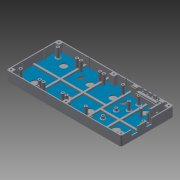
# Autodesk Inventor part: bottom-cover
Saved by Autodesk Inventor 2015 (Build 190159000, 159)
## iProperties
Created: 2016-04-25
Part Number: bottom-cover
Material: 一般
Document SubType Name: Modeling
Designer: yamashita1
Density: 1 g/cm^3
Appearance: 既定
Author: yamashita1
Autodesk Inventor part; units mm, degrees
ref_plane "YZ Plane" through (0, 0, 0) normal (1, 0, 0) x (0, 1, 0)
ref_plane "XZ Plane" through (0, 0, 0) normal (0, 1, 0) x (-1, 0, 0)
ref_plane "XY Plane" through (0, 0, 0) normal (0, 0, 1) x (1, 0, 0)
sketch "スケッチ1" plane through (0, 0, 0) normal (0, 0, 1) x (1, 0, 0)
  line L0 (-120, 55) -> (120, 55)
  line L1 (120, 55) -> (120, -55)
  line L2 (120, -55) -> (-120, -55)
  line L3 (-120, -55) -> (-120, 55)
  point P0 (0, 0)
  dimension "d0" = 240
  dimension "d1" = 110
  dimension "d2" = 120
  dimension "d3" = 55
  constraints: 8 end point, 2 parallel, 1 horizontal, 1 perpendicular
  measures "d0" distance of L1.end L2.end
  measures "d1" distance of L0.end L1.end
  measures "d2" distance from line of L3 point (0, 0)
  measures "d3" distance from line of L2 point (0, 0)
extrude "底" add sketch "スケッチ1" along normal blind 20
sketch "スケッチ2" plane through (0, 0, 20) normal (0, 0, 1) x (1, 0, 0)
  line L0 (-118, 53) -> (118, 53)
  line L1 (118, 53) -> (118, -53)
  line L2 (118, -53) -> (-118, -53)
  line L3 (-118, -53) -> (-118, 53)
  point P0 (0, 0)
  dimension "d6" = 236
  dimension "d7" = 106
  dimension "d8" = 118
  dimension "d9" = 53
  constraints: 8 end point, 2 parallel, 1 horizontal, 1 perpendicular
  measures "d6" distance of L1.end L2.end
  measures "d7" distance of L0.end L1.end
  measures "d8" distance from line of L3 point (0, 0)
  measures "d9" distance from line of L2 point (0, 0)
extrude "底 くりぬき" cut sketch "スケッチ2" against normal blind 18
sketch "スケッチ3" plane through (0, 0, 2) normal (0, 0, 1) x (1, 0, 0)
  line L0 (-118, 53) -> (-110, 53)
  line L1 (-110, 53) -> (-110, 45)
  line L2 (-110, 45) -> (-118, 45)
  line L3 (-118, 45) -> (-118, 53)
  line L4 (-118, -53) -> (-110, -53)
  line L5 (-110, -53) -> (-110, -45)
  line L6 (-110, -45) -> (-118, -45)
  line L7 (-118, -45) -> (-118, -53)
  line L8 (118, -53) -> (110, -53)
  line L9 (110, -53) -> (110, -45)
  line L10 (110, -45) -> (118, -45)
  line L11 (118, -45) -> (118, -53)
  line L12 (118, 53) -> (110, 53)
  line L13 (110, 53) -> (110, 45)
  line L14 (110, 45) -> (118, 45)
  line L15 (118, 45) -> (118, 53)
  line L16 (-5, 53) -> (5, 53)
  line L17 (5, 53) -> (5, 45)
  line L18 (5, 45) -> (-5, 45)
  line L19 (-5, 45) -> (-5, 53)
  line L20 (-5, -45) -> (5, -45)
  line L21 (5, -45) -> (5, -53)
  line L22 (5, -53) -> (-5, -53)
  line L23 (-5, -53) -> (-5, -45)
  line L24 (118, -53) -> (-118, -53) projected
  line L25 (-118, 53) -> (118, 53) projected
  point P0 (0, 0)
  point P1 (0, 45)
  point P2 (0, -53)
  point P3 (0, -53)
  point P4 (0, 53)
  dimension "d13" = 8
  dimension "d14" = 8
  dimension "d15" = 8
  dimension "d16" = 8
  dimension "d17" = 8
  dimension "d18" = 8
  dimension "d19" = 8
  dimension "d117" = 8
  dimension "d161" = 10
  dimension "d162" = 8
  dimension "d165" = 10
  dimension "d166" = 8
  constraints: 48 end point, 12 parallel, 6 horizontal, 6 perpendicular, 4 midpoint, 2 collinear, 2 vertical alignment, 1 coincident
  measures "d13" distance of L0.end L1.end
  measures "d14" distance of L6.end L5.end
  measures "d15" distance of L5.end L4.end
  measures "d16" distance of L9.end L10.end
  measures "d17" distance of L8.end L9.end
  measures "d18" distance of L14.end L13.end
  measures "d19" distance of L13.end L12.end
  measures "d117" distance from line of L3 L1.end
  measures "d161" distance of L17.end L18.end
  measures "d162" distance of L16.end L17.end
  measures "d165" distance of L21.end L22.end
  measures "d166" distance of L20.end L21.end
extrude "天板固定用ボス" add sketch "スケッチ3" along normal blind 18
sketch "スケッチ4" plane through (0, 0, 20) normal (0, 0, 1) x (1, 0, 0)
  circle A0 centre (-115, 50) radius 1.6
  line L0 (-120, 55) -> (-120, -55) projected
  line L1 (120, 55) -> (-120, 55) projected
  circle A1 centre (-115, -50) radius 1.6
  line L2 (-120, -55) -> (120, -55) projected
  circle A2 centre (115, 50) radius 1.6
  line L3 (120, -55) -> (120, 55) projected
  circle A3 centre (115, -50) radius 1.6
  circle A4 centre (0, 50) radius 1.6
  circle A5 centre (0, -50) radius 1.6
  point P0 (0, 0)
  dimension "d22" = 3.2
  dimension "d23" = 5
  dimension "d24" = 5
  dimension "d25" = 3.2
  dimension "d26" = 5
  dimension "d27" = 5
  dimension "d28" = 3.2
  dimension "d29" = 5
  dimension "d30" = 5
  dimension "d31" = 3.2
  dimension "d32" = 5
  dimension "d33" = 5
  constraints: 6 centre point, 2 equal radius, 2 horizontal alignment, 2 vertical alignment
  measures "d22" diameter of A0
  measures "d23" distance from line of L0 A0.centre
  measures "d24" distance from line of L1 A0.centre
  measures "d25" diameter of A1
  measures "d26" distance from line of L0 A1.centre
  measures "d27" distance from line of L2 A1.centre
  measures "d28" diameter of A2
  measures "d29" distance from line of L1 A2.centre
  measures "d30" distance from line of L3 A2.centre
  measures "d31" diameter of A3
  measures "d32" distance from line of L3 A3.centre
  measures "d33" distance from line of L2 A3.centre
extrude "天板固定用穴" cut sketch "スケッチ4" against normal blind 20 contours A0 | A1 | A2 | A3 | A4 | A5
sketch "スケッチ5" plane through (0, 0, 0) normal (0, 0, -1) x (-1, 0, 0)
  circle A0 centre (115, -50) radius 3.5
  circle A1 centre (115, -50) radius 1.6 projected
  circle A2 centre (115, 50) radius 3.5
  circle A3 centre (115, 50) radius 1.6 projected
  circle A4 centre (-115, 50) radius 3.5
  circle A5 centre (-115, 50) radius 1.6 projected
  circle A6 centre (-115, -50) radius 3.5
  circle A7 centre (-115, -50) radius 1.6 projected
  circle A8 centre (0, -50) radius 1.6 projected
  circle A9 centre (0, -50) radius 3.5
  circle A10 centre (0, 50) radius 1.6 projected
  circle A11 centre (0, 50) radius 3.5
  point P0 (0, 0)
  dimension "d39" = 7
  constraints: 6 centre point, 5 equal radius, 4 concentric, 2 coincident
  measures "d39" diameter of A6
extrude "天板固定用穴ザグリ" cut sketch "スケッチ5" against normal blind 15
sketch "スケッチ6" plane through (0, 0, 2) normal (0, 0, 1) x (1, 0, 0)
  circle A0 centre (-10, -39) radius 3.25
  circle A1 centre (-10, 39) radius 3.25
  circle A2 centre (30, 39) radius 3.25
  circle A3 centre (30, -39) radius 3.25
  point P0 (0, 0)
  dimension "d42" = 39
  dimension "d43" = 10
  dimension "d44" = 40
  dimension "d45" = 39
  dimension "d46" = 6.5
  dimension "d47" = 6.5
  dimension "d48" = 6.5
  dimension "d49" = 6.5
  constraints: 4 centre point, 4 coincident, 2 horizontal alignment, 2 vertical alignment
  measures "d42" vertical distance of point (-10, -39) point (0, 0)
  measures "d43" horizontal distance of point (-10, -39) point (0, 0)
  measures "d44" distance of point (30, -39) point (-10, -39)
  measures "d45" vertical distance of point (-10, 39) point (0, 0)
  measures "d46" diameter of A0
  measures "d47" diameter of A1
  measures "d48" diameter of A2
  measures "d49" diameter of A3
extrude "7セグ固定用ボス" add sketch "スケッチ6" along normal blind 19.4
sketch "スケッチ7" plane through (-10, 39, 21.4) normal (0, 0, 1) x (1, 0, 0)
  circle A0 centre (0, 0) radius 1.4
  circle A1 centre (0, 0) radius 3.25 projected
  circle A2 centre (0, -78) radius 1.4
  circle A3 centre (0, -78) radius 3.25 projected
  circle A4 centre (40, 0) radius 1.4
  circle A5 centre (40, 0) radius 3.25 projected
  circle A6 centre (40, -78) radius 1.4
  circle A7 centre (40, -78) radius 3.25 projected
  point P0 (10, -39)
  dimension "d52" = 2.8
  dimension "d53" = 2.8
  dimension "d54" = 2.8
  dimension "d55" = 2.8
  constraints: 4 centre point, 4 concentric
  measures "d52" diameter of A0
  measures "d53" diameter of A2
  measures "d54" diameter of A4
  measures "d55" diameter of A6
extrude "7セグ固定用ボス ねじ穴" cut sketch "スケッチ7" against normal blind 10 contours A0 | A2 | A4 | A6
pattern_linear "矩形状パターン1" count 3 spacing 48 along (-1, 0, 0) of "7セグ固定用ボス", "7セグ固定用ボス ねじ穴"
sketch "スケッチ8" plane through (120, -55, 0) normal (1, 0, 0) x (0, 0, -1)
  line L0 (-20, 110) -> (-20, 0) projected
  line L1 (-20, 53.38) -> (-9, 53.38)
  line L2 (-9, 53.38) -> (-9, 64.38)
  line L3 (-9, 64.38) -> (-20, 64.38)
  line L4 (-20, 64.38) -> (-20, 53.38)
  line L5 (-20, 21.9) -> (-9, 21.9)
  line L6 (-9, 21.9) -> (-9, 34.9)
  line L7 (-9, 34.9) -> (-20, 34.9)
  line L8 (-20, 34.9) -> (-20, 21.9)
  line L9 (-20, 0) -> (-20, 110) projected
  point P0 (0, 55)
  point P1 (-20, 66.5)
  point P2 (-20, 58.88)
  point P3 (-20, 28.4)
  point P4 (-20, 58.88)
  point P5 (-20, 28.4)
  dimension "d197" = 11.5
  dimension "d198" = 7.62
  dimension "d199" = 38.1
  dimension "d200" = 11
  dimension "d201" = 11
  dimension "d202" = 11
  dimension "d203" = 13
  constraints: 16 end point, 4 parallel, 3 point on line, 2 coincident, 2 collinear, 2 horizontal, 2 midpoint, 2 perpendicular
  measures "d197" vertical distance of point (0, 55) point (-20, 66.5)
  measures "d198" distance of point (-20, 58.88) point (-20, 66.5)
  measures "d199" distance of point (-20, 28.4) point (-20, 66.5)
  measures "d200" distance of L3.end L2.end
  measures "d201" distance of L2.end L1.end
  measures "d202" distance of L7.end L6.end
  measures "d203" distance of L6.end L5.end
extrude "Arduinoコネクタ穴" cut sketch "スケッチ8" against normal blind 2
sketch "スケッチ9" plane through (0, 0, 2) normal (0, 0, 1) x (1, 0, 0)
  line L0 (118, 45) -> (118, -45) projected
  circle A0 centre (103.03, 8.96) radius 3
  circle A1 centre (50.96, 3.88) radius 3
  circle A2 centre (50.96, -24.06) radius 3
  circle A3 centre (101.76, -39.3) radius 3
  point P0 (0, 0)
  point P1 (118, 11.5)
  point P2 (118, 8.88)
  dimension "d75" = 11.5
  dimension "d76" = 14.97
  dimension "d77" = 2.54
  dimension "d78" = 67.04
  dimension "d79" = 7.62
  dimension "d80" = 27.94
  dimension "d81" = 16.24
  dimension "d82" = 50.8
  dimension "d83" = 6
  constraints: 4 centre point, 4 coincident, 3 equal radius, 1 point on line, 1 vertical alignment
  measures "d75" vertical distance of point (118, 11.5) point (0, 0)
  measures "d76" horizontal distance of point (103.03, 8.96) point (118, 11.5)
  measures "d77" vertical distance of point (103.03, 8.96) point (118, 11.5)
  measures "d78" horizontal distance of point (50.96, 3.88) point (118, 11.5)
  measures "d79" vertical distance of point (50.96, 3.88) point (118, 11.5)
  measures "d80" distance of point (50.96, -24.06) point (50.96, 3.88)
  measures "d81" horizontal distance of point (101.76, -39.3) point (118, 11.5)
  measures "d82" vertical distance of point (101.76, -39.3) point (118, 11.5)
  measures "d83" diameter of A0
extrude "Arduino固定用ボス" add sketch "スケッチ9" along normal blind 5.2
sketch "スケッチ10" plane through (103.03, 8.96, 7.2) normal (0, 0, 1) x (1, 0, 0)
  circle A0 centre (0, 0) radius 1.4
  circle A1 centre (0, 0) radius 3 projected
  circle A2 centre (-52.07, -5.08) radius 1.4
  circle A3 centre (-52.07, -33.02) radius 1.4
  circle A4 centre (-52.07, -5.08) radius 3 projected
  circle A5 centre (-52.07, -33.02) radius 3 projected
  point P0 (-103.03, -8.96)
  dimension "d86" = 2.8
  constraints: 3 centre point, 3 concentric, 2 equal radius
  measures "d86" diameter of A0
extrude "Arduino固定用ボス ねじ穴" cut sketch "スケッチ10" against normal blind 5.2 contours A0 | A2 | A3
sketch "スケッチ11" plane through (-120, 55, 0) normal (0, 1, 0) x (1, 0, 0)
  line L0 (230, -20) -> (10, -20) projected
  line L1 (209.24, -20) -> (205.24, -20)
  line L2 (205.24, -20) -> (205.24, -14.5)
  line L3 (205.24, -14.5) -> (209.24, -14.5)
  line L4 (209.24, -14.5) -> (209.24, -20)
  line L5 (240, -20) -> (0, -20) projected
  point P0 (120, 0)
  point P1 (192, -20)
  point P2 (207.24, -20)
  point P3 (207.24, -14.5)
  dimension "d89" = 72
  dimension "d90" = 15.24
  dimension "d91" = 4
  dimension "d92" = 5.5
  constraints: 8 end point, 2 parallel, 2 point on line, 1 collinear, 1 horizontal, 1 midpoint, 1 perpendicular, 1 vertical alignment
  measures "d89" horizontal distance of point (192, -20) point (120, 0)
  measures "d90" distance of point (207.24, -20) point (192, -20)
  measures "d91" distance of L2.end L3.end
  measures "d92" distance of L1.end L2.end
extrude "タクトスイッチ穴" cut sketch "スケッチ11" against normal blind 2
pattern_linear "矩形状パターン2" count 4 spacing 10.16 along (-1, 0, 0) of "タクトスイッチ穴"
sketch "スケッチ12" plane through (0, 0, 2) normal (0, 0, 1) x (1, 0, 0)
  line L0 (-110, 53) -> (110, 53) projected
  line L1 (40, 53) -> (104, 53)
  line L2 (104, 53) -> (104, 45)
  line L3 (104, 45) -> (40, 45)
  line L4 (40, 45) -> (40, 53)
  line L5 (68.92, 53) -> (75.08, 53) projected
  line L6 (89.24, 53) -> (110, 53) projected
  point P0 (0, 0)
  point P1 (72, 53)
  point P2 (72, 45)
  point P3 (72, 53)
  dimension "d98" = 72
  dimension "d99" = 64
  dimension "d100" = 8
  constraints: 8 end point, 2 midpoint, 2 parallel, 1 collinear, 1 horizontal, 1 perpendicular, 1 point on line, 1 vertical alignment
  measures "d98" horizontal distance of point (72, 53) point (0, 0)
  measures "d99" distance of L2.end L3.end
  measures "d100" distance of L1.end L2.end
extrude "タクトスイッチ固定用ボス" add sketch "スケッチ12" along normal blind 18
sketch "スケッチ13" plane through (0, 0, 20) normal (0, 0, 1) x (1, 0, 0)
  line L0 (75.08, 55) -> (68.92, 55) projected
  line L1 (42, 48) -> (102, 48)
  line L2 (102, 48) -> (102, 46.2)
  line L3 (102, 46.2) -> (42, 46.2)
  line L4 (42, 46.2) -> (42, 48)
  point P0 (0, 0)
  point P1 (72, 55)
  point P2 (72, 46.2)
  point P3 (72, 55)
  dimension "d103" = 60
  dimension "d104" = 1.8
  dimension "d105" = 7
  constraints: 8 end point, 3 midpoint, 2 parallel, 1 horizontal, 1 perpendicular, 1 vertical alignment
  measures "d103" distance of L2.end L3.end
  measures "d104" distance of L1.end L2.end
  measures "d105" vertical distance of L1.start point (72, 55)
extrude "タクトスイッチ基板用スリット" cut sketch "スケッチ13" against normal blind 11
sketch "スケッチ14" plane through (0, 0, 20) normal (0, 0, 1) x (1, 0, 0)
  line L0 (75.08, 55) -> (68.92, 55) projected
  line L1 (49.5, 53) -> (94.5, 53)
  line L2 (94.5, 53) -> (94.5, 48)
  line L3 (94.5, 48) -> (49.5, 48)
  line L4 (49.5, 48) -> (49.5, 53)
  point P0 (0, 0)
  point P1 (72, 55)
  point P2 (72, 48)
  point P3 (72, 55)
  dimension "d108" = 45
  dimension "d109" = 5
  dimension "d110" = 2
  constraints: 8 end point, 3 midpoint, 2 parallel, 1 horizontal, 1 perpendicular, 1 vertical alignment
  measures "d108" distance of L2.end L3.end
  measures "d109" distance of L1.end L2.end
  measures "d110" vertical distance of L1.start point (72, 55)
extrude "タクトスイッチ基板用くりぬき1" cut sketch "スケッチ14" against normal blind 6.8
sketch "スケッチ15" plane through (0, 0, 20) normal (0, 0, 1) x (1, 0, 0)
  line L0 (75.08, 55) -> (68.92, 55) projected
  line L1 (49.5, 45) -> (94.5, 45)
  line L2 (94.5, 45) -> (94.5, 47.5)
  line L3 (94.5, 47.5) -> (49.5, 47.5)
  line L4 (49.5, 47.5) -> (49.5, 45)
  line L5 (40, 45) -> (104, 45) projected
  point P0 (0, 0)
  point P1 (72, 55)
  point P2 (72, 45)
  point P3 (72, 55)
  dimension "d113" = 45
  dimension "d114" = 2.5
  constraints: 8 end point, 3 midpoint, 2 parallel, 1 collinear, 1 horizontal, 1 perpendicular, 1 vertical alignment
  measures "d113" distance of L3.end L2.end
  measures "d114" distance of L2.end L1.end
extrude "タクトスイッチ基板用くりぬき2" cut sketch "スケッチ15" against normal blind 7.5
sketch "スケッチ16" plane through (0, 0, 2) normal (0, 0, 1) x (1, 0, 0)
  circle A0 centre (104.32, 38.16) radius 3
  circle A1 centre (63.68, 38.16) radius 3
  circle A2 centre (63.68, 17.84) radius 3
  circle A3 centre (104.32, 17.84) radius 3
  circle A4 centre (89.08, 17.84) radius 2.5
  point P0 (0, 0)
  point P1 (84, 28)
  dimension "d118" = 84
  dimension "d119" = 28
  dimension "d120" = 20.32
  dimension "d121" = 10.16
  dimension "d122" = 20.32
  dimension "d123" = 10.16
  dimension "d124" = 6
  dimension "d125" = 5.08
  dimension "d126" = 5
  constraints: 5 centre point, 5 coincident, 3 equal radius, 3 horizontal alignment, 2 vertical alignment
  measures "d118" horizontal distance of point (84, 28) point (0, 0)
  measures "d119" vertical distance of point (0, 0) point (84, 28)
  measures "d120" horizontal distance of point (104.32, 38.16) point (84, 28)
  measures "d121" vertical distance of point (84, 28) point (104.32, 38.16)
  measures "d122" horizontal distance of point (84, 28) point (63.68, 38.16)
  measures "d123" vertical distance of point (104.32, 17.84) point (84, 28)
  measures "d124" diameter of A0
  measures "d125" horizontal distance of point (84, 28) point (89.08, 17.84)
  measures "d126" diameter of A4
extrude "LCD RTC基板固定用ボス" add sketch "スケッチ16" along normal blind 16.7
sketch "スケッチ17" plane through (104.32, 38.16, 18.7) normal (0, 0, 1) x (1, 0, 0)
  circle A0 centre (0, 0) radius 1.4
  circle A1 centre (-40.64, 0) radius 1.4
  circle A2 centre (-40.64, -20.32) radius 1.4
  circle A3 centre (0, -20.32) radius 1.4
  circle A4 centre (0, 0) radius 3 projected
  circle A5 centre (-40.64, 0) radius 3 projected
  circle A6 centre (-40.64, -20.32) radius 3 projected
  circle A7 centre (0, -20.32) radius 3 projected
  point P0 (-104.32, -38.16)
  dimension "d129" = 2.8
  constraints: 4 centre point, 4 concentric, 3 equal radius
  measures "d129" diameter of A0
extrude "LCD RTC基板固定用ボス ねじ穴" cut sketch "スケッチ17" against normal blind 10 contours A0 | A1 | A2 | A3
sketch "スケッチ18" plane through (0, 0, 2) normal (0, 0, 1) x (1, 0, 0)
  line L0 (110.5, 37.96) -> (113.5, 37.96)
  line L1 (113.5, 37.96) -> (113.5, 12.96)
  line L2 (113.5, 12.96) -> (110.5, 12.96)
  line L3 (110.5, 12.96) -> (110.5, 37.96)
  point P0 (0, 0)
  point P1 (84, 28)
  point P2 (113.5, 25.46)
  point P3 (112, 12.96)
  point P4 (112, 25.46)
  dimension "d132" = 84
  dimension "d133" = 28
  dimension "d135" = 3
  dimension "d136" = 25
  dimension "d204" = 2.54
  dimension "d205" = 28
  constraints: 8 end point, 2 midpoint, 2 parallel, 1 horizontal, 1 horizontal alignment, 1 perpendicular, 1 vertical alignment
  measures "d132" horizontal distance of point (84, 28) point (0, 0)
  measures "d133" vertical distance of point (84, 28) point (0, 0)
  measures "d135" distance of L1.end L2.end
  measures "d136" distance of L0.end L1.end
  measures "d204" vertical distance of point (84, 28) point (112, 25.46)
  measures "d205" horizontal distance of point (84, 28) point (112, 25.46)
extrude "LCD支持用ボス" add sketch "スケッチ18" along normal blind 29.5
sketch "スケッチ22" plane through (0, 0, 31.5) normal (0, 0, 1) x (1, 0, 0)
  line L0 (110.5, 12.96) -> (110.5, 37.96) projected
  line L1 (113.5, 12.96) -> (113.5, 37.96) projected
  line L2 (110.5, 36.71) -> (113.5, 36.71)
  line L3 (113.5, 36.71) -> (113.5, 14.21)
  line L4 (113.5, 14.21) -> (110.5, 14.21)
  line L5 (110.5, 14.21) -> (110.5, 36.71)
  point P0 (0, 0)
  point P1 (113.5, 25.46)
  point P2 (113.5, 25.46)
  dimension "d206" = 22.5
  constraints: 8 end point, 2 midpoint, 2 parallel, 2 point on line, 1 coincident, 1 horizontal, 1 perpendicular
  measures "d206" distance of L2.end L3.end
extrude "LCD支持用ボス くぼみ" cut sketch "スケッチ22" against normal blind 1
fillet "フィレット1" radius 3 4 edges at (120, -55, 10) (120, 55, 10) (-120, -55, 10) (-120, 55, 10)
sketch "スケッチ19" plane through (0, 0, 2) normal (0, 0, 1) x (1, 0, 0)
  circle A0 centre (-45, 25) radius 5
  circle A1 centre (45, 25) radius 5
  circle A2 centre (-45, 33) radius 2
  circle A3 centre (45, 33) radius 2
  line L0 (-47, 33) -> (-43, 33)
  line L1 (-43, 33) -> (-43, 29)
  line L2 (-43, 29) -> (-47, 29)
  line L3 (-47, 29) -> (-47, 33)
  line L4 (43, 33) -> (47, 33)
  line L5 (47, 33) -> (47, 29)
  line L6 (47, 29) -> (43, 29)
  line L7 (43, 29) -> (43, 33)
  point P0 (0, 0)
  dimension "d146" = 4
  dimension "d147" = 4
  dimension "d140" = 25
  dimension "d141" = 45
  dimension "d142" = 45
  dimension "d143" = 10
  dimension "d144" = 10
  dimension "d145" = 8
  dimension "d148" = 4
  dimension "d149" = 4
  dimension "d150" = 4
  dimension "d151" = 4
  constraints: 16 end point, 6 coincident, 4 horizontal alignment, 4 parallel, 2 centre point, 2 horizontal, 2 midpoint, 2 perpendicular, 2 vertical alignment, 4 other
  measures "d140" vertical distance of point (-45, 25) point (0, 0)
  measures "d141" horizontal distance of point (-45, 25) point (0, 0)
  measures "d142" horizontal distance of point (45, 25) point (0, 0)
  measures "d143" diameter of A0
  measures "d144" diameter of A1
  measures "d145" distance of point (-45, 33) A0.centre
  measures "d148" distance of L1.end L2.end
  measures "d149" distance of L0.end L1.end
  measures "d150" distance of L5.end L6.end
  measures "d151" distance of L4.end L5.end
extrude "壁掛けねじ穴" cut sketch "スケッチ19" against normal blind 2
sketch "スケッチ20" plane through (0, 0, 2) normal (0, 0, 1) x (1, 0, 0)
  circle A0 centre (85, 30) radius 7
  circle A1 centre (-85, 30) radius 7
  circle A2 centre (-85, -30) radius 7
  circle A3 centre (85, -30) radius 7
  circle A4 centre (24, 24) radius 7
  circle A5 centre (-24, 24) radius 7
  circle A6 centre (24, -24) radius 7
  circle A7 centre (-24, -24) radius 7
  point P0 (0, 0)
  dimension "d154" = 30
  dimension "d155" = 85
  dimension "d156" = 85
  dimension "d157" = 30
  dimension "d158" = 14
  dimension "d167" = 24
  dimension "d168" = 24
  dimension "d169" = 24
  dimension "d170" = 24
  constraints: 8 centre point, 8 coincident, 7 equal radius, 4 horizontal alignment, 4 vertical alignment
  measures "d154" vertical distance of point (85, 30) point (0, 0)
  measures "d155" horizontal distance of point (85, 30) point (0, 0)
  measures "d156" horizontal distance of point (-85, 30) point (0, 0)
  measures "d157" vertical distance of point (85, -30) point (0, 0)
  measures "d158" diameter of A0
  measures "d167" horizontal distance of point (24, 24) point (0, 0)
  measures "d168" horizontal distance of point (24, 24) point (0, 0)
  measures "d169" horizontal distance of point (-24, 24) point (0, 0)
  measures "d170" horizontal distance of point (24, -24) point (0, 0)
extrude "磁石用くぼみ" cut sketch "スケッチ20" against normal blind 1.7
sketch "スケッチ21" plane through (0, 0, 2) normal (0, 0, 1) x (1, 0, 0)
  line L0 (-118, -45) -> (-118, 45) projected
  line L1 (120, 52) -> (120, -52) projected
  line L2 (118, 45) -> (118, -45) projected
  line L3 (-5, -53) -> (-110, -53) projected
  line L4 (110, -53) -> (5, -53) projected
  line L5 (-110, 53) -> (-5, 53) projected
  line L6 (-116, 25) -> (-118, 25)
  line L7 (-118, 25) -> (-118, 21)
  line L8 (-118, 21) -> (-116, 21)
  line L9 (-116, 21) -> (-116, 25)
  line L10 (-118, -45) -> (-118, 45) projected
  line L11 (-118, -21) -> (-116, -21)
  line L12 (-116, -21) -> (-116, -25)
  line L13 (-116, -25) -> (-118, -25)
  line L14 (-118, -25) -> (-118, -21)
  line L15 (-57, -51) -> (-53, -51)
  line L16 (-53, -51) -> (-53, -53)
  line L17 (-53, -53) -> (-57, -53)
  line L18 (-57, -53) -> (-57, -51)
  line L19 (-5, -53) -> (-110, -53) projected
  line L20 (53, -51) -> (57, -51)
  line L21 (57, -51) -> (57, -53)
  line L22 (57, -53) -> (53, -53)
  line L23 (53, -53) -> (53, -51)
  line L24 (110, -53) -> (5, -53) projected
  line L25 (-57, 53) -> (-53, 53)
  line L26 (-53, 53) -> (-53, 51)
  line L27 (-53, 51) -> (-57, 51)
  line L28 (-57, 51) -> (-57, 53)
  line L29 (-110, 53) -> (-5, 53) projected
  line L30 (5, 53) -> (40, 53) projected
  line L31 (24.5, 51) -> (20.5, 51)
  line L32 (20.5, 51) -> (20.5, 53)
  line L33 (20.5, 53) -> (24.5, 53)
  line L34 (24.5, 53) -> (24.5, 51)
  line L35 (116, 25) -> (118, 25)
  line L36 (118, 25) -> (118, 21)
  line L37 (118, 21) -> (116, 21)
  line L38 (116, 21) -> (116, 25)
  line L39 (118, 45) -> (118, -45) projected
  point P0 (0, 0)
  point P1 (-118, 23)
  point P2 (-118, -23)
  point P3 (118, 23)
  point P4 (-55, -53)
  point P5 (55, -53)
  point P6 (-55, 53)
  point P7 (-118, 23)
  point P8 (-118, -23)
  point P9 (-55, -53)
  point P10 (55, -53)
  point P11 (-55, 53)
  point P12 (22.5, 53)
  point P13 (22.5, 53)
  point P14 (22.5, 53)
  point P15 (118, 23)
  point P16 (118, 8.88)
  dimension "d171" = 23
  dimension "d172" = 23
  dimension "d173" = 55
  dimension "d174" = 55
  dimension "d175" = 2
  dimension "d176" = 4
  dimension "d177" = 4
  dimension "d178" = 2
  dimension "d179" = 4
  dimension "d180" = 2
  dimension "d181" = 4
  dimension "d182" = 2
  dimension "d183" = 4
  dimension "d184" = 2
  dimension "d185" = 4
  dimension "d186" = 2
  dimension "d187" = 4
  dimension "d188" = 2
  constraints: 56 end point, 14 parallel, 9 midpoint, 7 coincident, 7 collinear, 7 horizontal, 7 perpendicular, 6 point on line, 1 horizontal alignment, 1 vertical alignment
  measures "d171" vertical distance of point (-118, 23) point (0, 0)
  measures "d172" vertical distance of point (-118, -23) point (0, 0)
  measures "d173" horizontal distance of point (-55, -53) point (0, 0)
  measures "d174" horizontal distance of point (55, -53) point (0, 0)
  measures "d175" distance of L8.end L7.end
  measures "d176" distance of L7.end L6.end
  measures "d177" distance of L11.end L12.end
  measures "d178" distance of L12.end L13.end
  measures "d179" distance of L15.start L15.end
  measures "d180" distance of L17.end L15.start
  measures "d181" distance of L20.start L20.end
  measures "d182" distance of L22.end L20.start
  measures "d183" distance of L26.end L27.end
  measures "d184" distance of L27.end L25.start
  measures "d185" distance of L31.start L31.end
  measures "d186" distance of L31.end L32.end
  measures "d187" distance of L37.end L35.start
  measures "d188" distance of L36.end L37.end
extrude "位置合わせ爪" add sketch "スケッチ21" along normal blind 20
fillet "フィレット2" radius 2 9 edges at (47.96, 3.88, 2) (47.96, -24.06, 2) (100.03, 8.96, 2) (60.68, 38.16, 2) (60.68, 17.84, 2) (101.32, 17.84, 2) (101.32, 38.16, 2) (-109.25, 39, 2) (-109.25, -39, 2)
sketch "スケッチ23" plane through (0, 0, 2) normal (0, 0, 1) x (1, 0, 0)
  line L0 (24.5, 53) -> (40, 53) projected
  line L1 (53, -53) -> (5, -53) projected
  line L2 (36, 53) -> (32, 53)
  line L3 (32, 53) -> (32, -53)
  line L4 (32, -53) -> (36, -53)
  line L5 (36, -53) -> (36, 53)
  line L6 (-53, 53) -> (-5, 53) projected
  line L7 (-5, -53) -> (-53, -53) projected
  line L8 (-16, 53) -> (-12, 53)
  line L9 (-12, 53) -> (-12, -53)
  line L10 (-12, -53) -> (-16, -53)
  line L11 (-16, -53) -> (-16, 53)
  line L12 (-110, 53) -> (-57, 53) projected
  line L13 (-57, -53) -> (-110, -53) projected
  line L14 (-64, 53) -> (-60, 53)
  line L15 (-60, 53) -> (-60, -53)
  line L16 (-60, -53) -> (-64, -53)
  line L17 (-64, -53) -> (-64, 53)
  line L18 (-118, -21) -> (-118, 21) projected
  line L19 (-118, 2) -> (32, 2)
  line L20 (32, 2) -> (32, -2)
  line L21 (32, -2) -> (-118, -2)
  line L22 (-118, -2) -> (-118, 2)
  line L23 (118, -1.62) -> (118, -20.1) projected
  line L24 (118, -10) -> (36, -10)
  line L25 (36, -10) -> (36, -14)
  line L26 (36, -14) -> (118, -14)
  line L27 (118, -14) -> (118, -10)
  line L28 (110, -53) -> (57, -53) projected
  line L29 (72, 44.8085) -> (76, 44.8085)
  line L30 (76, 44.8085) -> (76, -53)
  line L31 (76, -53) -> (72, -53)
  line L32 (72, -53) -> (72, 44.8085)
  point P0 (0, 0)
  point P1 (34, 0)
  point P2 (34, 53)
  point P3 (-14, 0)
  point P4 (-62, 0)
  point P5 (-14, 53)
  point P6 (-62, 53)
  point P7 (32, 0)
  point P8 (34, -12)
  point P9 (36, -12)
  point P10 (74, -12)
  point P11 (74, 44.8085)
  dimension "d210" = 34
  dimension "d211" = 4
  dimension "d212" = 48
  dimension "d213" = 48
  dimension "d214" = 4
  dimension "d215" = 4
  dimension "d216" = 4
  dimension "d217" = 12
  dimension "d218" = 4
  dimension "d219" = 40
  dimension "d220" = 4
  constraints: 48 end point, 12 parallel, 11 point on line, 6 horizontal, 6 horizontal alignment, 6 midpoint, 6 perpendicular, 5 vertical alignment
  measures "d210" distance of point (0, 0) point (34, 0)
  measures "d211" distance of L4.end L3.end
  measures "d212" distance of point (-14, 0) point (34, 0)
  measures "d213" distance of point (-62, 0) point (-14, 0)
  measures "d214" distance of L9.end L10.end
  measures "d215" distance of L15.end L16.end
  measures "d216" distance of L20.end L19.end
  measures "d217" distance of point (34, -12) point (34, 0)
  measures "d218" distance of L25.end L24.end
  measures "d219" distance of point (74, -12) point (34, -12)
  measures "d220" distance of L30.end L31.end
extrude "底面 補強材" add sketch "スケッチ23" along normal blind 3
equation "\"d2\" = 0.5 * d0"
equation "\"d3\" = 0.5 * d1"
equation "\"d8\" = 0.5 * d6"
equation "\"d9\" = 0.5 * d7"
equation "\"d45\" = d42"
equation "\"d122\" = d120"
equation "\"d123\" = d121"
equation "\"d142\" = d141"
equation "\"d156\" = d155"
equation "\"d157\" = d154"
equation "\"d169\" = d167"
equation "\"d170\" = d168"
equation "\"d172\" = d171"
equation "\"d174\" = d173"
equation "\"d177\" = d176"
equation "\"d178\" = d175"
equation "\"d179\" = d177"
equation "\"d180\" = d178"
equation "\"d181\" = d179"
equation "\"d182\" = d180"
equation "\"d183\" = d176"
equation "\"d184\" = d175"
equation "\"d185\" = d183"
equation "\"d186\" = d184"
equation "\"d187\" = d185"
equation "\"d188\" = d186"
equation "\"d214\" = d211"
equation "\"d215\" = d211"
equation "\"d216\" = d211"
equation "\"d218\" = d211"
equation "\"d220\" = d211"
